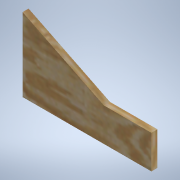
# Autodesk Inventor part: Sides
Saved by Autodesk Inventor 2021.1 (Build 251245000, 245)
## iProperties
Created: 2020-08-02
Part Number: Sides
Material: Generic
Document SubType Name: Modeling
Designer: adick
Density: 1 g/cm^3
Appearance: Default
Author: adick
Autodesk Inventor part; units mm, degrees
ref_plane "YZ Plane" through (0, 0, 0) normal (1, 0, 0) x (0, 1, 0)
ref_plane "XZ Plane" through (0, 0, 0) normal (0, 1, 0) x (-1, 0, 0)
ref_plane "XY Plane" through (0, 0, 0) normal (0, 0, 1) x (1, 0, 0)
sketch "Sketch1" plane through (0, 0, 0) normal (0, 0, 1) x (1, 0, 0)
  line L0 (-270, 1) -> (-270, 72)
  line L1 (-99.577, 71) -> (0, 71)
  line L2 (0, 71) -> (0, 0)
  line L3 (-99.577, 71) -> (-270, 155)
  line L4 (-270, 155) -> (-270, 72)
  line L5 (0, 1) -> (0, -5.35)
  line L6 (0, -5.35) -> (-270, -5.35)
  line L7 (-270, -5.35) -> (-270, 1)
  line L8 (0, -5.35) -> (-270, -5.35) projected
  point P0 (0, 0)
  constraints: 16 end point, 2 parallel
extrude "Extrusion1" add sketch "Sketch1" along normal blind 12.7
body "Solid1"
